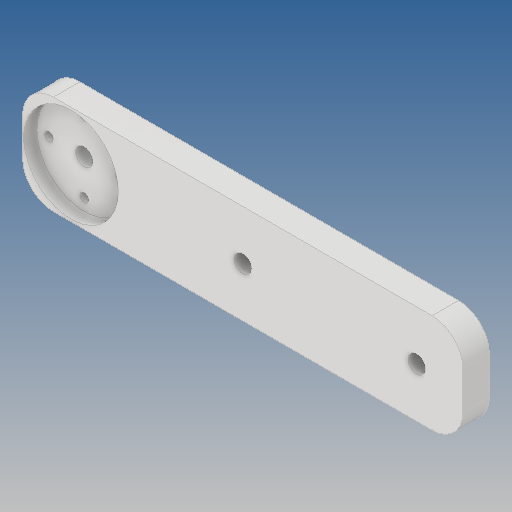
# Autodesk Inventor part: peregorodka
Saved by Autodesk Inventor 2020 (Build 240168000, 168)
## iProperties
Created: 2019-08-29
Part Number: peregorodka
Material: Пластик АБС
Document SubType Name: Modeling
Designer: Professional
Density: 1.06 g/cm^3
Appearance: Гладкий — белый
Author: Professional
Autodesk Inventor part; units mm, degrees
ref_plane "YZ Plane" through (0, 0, 0) normal (1, 0, 0) x (0, 1, 0)
ref_plane "XZ Plane" through (0, 0, 0) normal (0, 1, 0) x (-1, 0, 0)
ref_plane "XY Plane" through (0, 0, 0) normal (0, 0, 1) x (1, 0, 0)
sketch "Эскиз1" plane through (0, 0, 0) normal (0, 0, 1) x (1, 0, 0)
  line L0 (0, 0) -> (-100, 0)
  line L1 (-100, 0) -> (-100, 22.5)
  line L2 (-100, 22.5) -> (0, 22.5)
  line L3 (0, 22.5) -> (0, 0)
  line L4 (-100, 11.25) -> (0, 11.25) construction
  line L5 (0, 11.25) -> (-10.5, 11.25) construction
  circle A0 centre (-10.5, 11.25) radius 10.5 construction
  circle A1 centre (-89, 11.25) radius 10.75
  line L6 (-50, 0) -> (-50, 22.5) construction
  circle A2 centre (-50, 11.25) radius 2
  circle A3 centre (-10.5, 11.25) radius 2
  dimension "d0" = 100
  dimension "d1" = 22.5
  dimension "d2" = 10.5
  dimension "d3" = 11
  dimension "d4" = 21
  dimension "d5" = 21.5
  dimension "d6" = 4
  dimension "d7" = 4
  constraints: 14 end point, 5 midpoint, 4 centre point, 2 coincident, 2 parallel, 1 horizontal, 1 perpendicular, 1 point on line
  measures "d0" distance of L0.start L0.end
  measures "d1" distance of L2.end L0.start
  measures "d2" distance of L4.end L5.end
  measures "d3" distance of L4.start A1.centre
  measures "d4" diameter of A0
  measures "d5" diameter of A1
  measures "d6" diameter of A2
  measures "d7" diameter of A3
extrude "Выдавливание1" add sketch "Эскиз1" along normal blind 6
sketch "Эскиз2" plane through (0, 0, 0) normal (0, 0, -1) x (-1, 0, 0)
  circle A0 centre (89, 11.25) radius 10.75 projected
  circle A1 centre (89, 11.25) radius 10.75
  point P0 (0, 0)
  point P1 (89.5, 21)
  point P2 (89.5, 0)
  dimension "d23" = 21.5
  constraints: 1 centre point, 1 coincident, 1 other
  measures "d23" diameter of A1
extrude "Выдавливание2" add sketch "Эскиз2" against normal blind 3
sketch "Эскиз3" plane through (0, 0, 3) normal (0, 0, 1) x (1, 0, 0)
  circle A0 centre (-89, 11.25) radius 10.75 projected
  circle A1 centre (-89, 11.25) radius 2
  point P0 (0, 0)
  point P1 (-89.5, 21)
  point P2 (-89.5, 0)
  dimension "d12" = 4
  constraints: 1 centre point, 1 coincident, 1 other
  measures "d12" diameter of A1
extrude "Выдавливание3" cut sketch "Эскиз3" against normal blind 3 contours A1
fillet "Сопряжение1" radius 7 4 edges at (0, 22.5, 3) (0, 0, 3) (-100, 22.5, 3) (-100, 0, 3)
sketch "Эскиз4" plane through (0, 0, 0) normal (0, 0, -1) x (-1, 0, 0)
  circle A0 centre (89, 11.25) radius 2 projected
  circle A1 centre (89, 11.25) radius 8 construction
  circle A2 centre (81, 11.25) radius 1
  circle A3 centre (89, 3.25) radius 1
  circle A4 centre (97, 11.25) radius 1
  circle A5 centre (89, 19.25) radius 1
  point P0 (0, 0)
  dimension "d16" = 16
  dimension "d17" = 2
  dimension "d18" = 2
  dimension "d19" = 2
  dimension "d20" = 2
  constraints: 5 centre point, 4 point on circle, 2 horizontal alignment, 2 vertical alignment, 1 coincident
  measures "d16" diameter of A1
  measures "d17" diameter of A2
  measures "d18" diameter of A3
  measures "d19" diameter of A4
  measures "d20" diameter of A5
extrude "Выдавливание4" cut sketch "Эскиз4" against normal blind 6 contours A2 | A3 | A4 | A5
